Autodesk Fusion 360 part; units mm, degrees
note: some values were not read from the file. Set by a fixed rule: which face or edge a step refers to.
(part 2 of 2)
sketch "Sketch12" plane through (0, 3, 0) normal (0, 1, 0) x (-1, 0, 0) in component "DisplayMount"
  circle A0 centre (-31.9526, 89.8787) radius 5.5
  circle A1 centre (-31.9526, 43.8787) radius 5.5
  circle A2 centre (-230, 35) radius 6.5
  circle A3 centre (-230, 113) radius 6.5
  circle A4 centre (-204.5, 33.25) radius 0.95
  circle A5 centre (-254, 101.75) radius 0.95
  circle A6 centre (-204.5, 101.75) radius 0.95
  circle A7 centre (-254, 33.25) radius 0.95
  line L0 (-205.5, 60.85) -> (-205.5, 66.5)
  line L1 (-205.5, 66.5) -> (-196.5, 66.5)
  line L2 (-196.5, 66.5) -> (-196.5, 60.85)
  line L3 (-196.5, 60.85) -> (-205.5, 60.85)
  line L4 (-205.5, 129.35) -> (-205.5, 135)
  line L5 (-205.5, 135) -> (-196.5, 135)
  line L6 (-196.5, 135) -> (-196.5, 129.35)
  line L7 (-196.5, 129.35) -> (-205.5, 129.35)
  line L8 (-262, 68.5) -> (-262, 74.15)
  line L9 (-262, 74.15) -> (-252.75, 74.15)
  line L10 (-252.75, 74.15) -> (-252.75, 68.5)
  line L11 (-252.75, 68.5) -> (-262, 68.5)
  line L12 (-262, 0) -> (-262, 5.65)
  line L13 (-262, 5.65) -> (-252.75, 5.65)
  line L14 (-252.75, 5.65) -> (-252.75, 0)
  line L15 (-252.75, 0) -> (-262, 0)
  circle A8 centre (-139, 33.25) radius 0.95
  circle A9 centre (-188.5, 101.75) radius 0.95
  circle A10 centre (-139, 101.75) radius 0.95
  line L16 (-140, 60.85) -> (-140, 66.5)
  line L17 (-140, 66.5) -> (-131, 66.5)
  line L18 (-131, 66.5) -> (-131, 60.85)
  line L19 (-131, 60.85) -> (-140, 60.85)
  line L20 (-140, 129.35) -> (-140, 135)
  line L21 (-140, 135) -> (-131, 135)
  line L22 (-131, 135) -> (-131, 129.35)
  line L23 (-131, 129.35) -> (-140, 129.35)
  line L24 (-196.5, 68.5) -> (-196.5, 74.15)
  line L25 (-196.5, 74.15) -> (-187.25, 74.15)
  line L26 (-187.25, 74.15) -> (-187.25, 68.5)
  line L27 (-187.25, 68.5) -> (-196.5, 68.5)
  line L28 (-196.5, 0) -> (-196.5, 5.65)
  line L29 (-196.5, 5.65) -> (-187.25, 5.65)
  line L30 (-187.25, 5.65) -> (-187.25, 0)
  line L31 (-187.25, 0) -> (-196.5, 0)
  circle A11 centre (-73.5, 33.25) radius 0.95
  circle A12 centre (-123, 101.75) radius 0.95
  circle A13 centre (-73.5, 101.75) radius 0.95
  circle A14 centre (-123, 33.25) radius 0.95
  line L32 (-74.5, 60.85) -> (-74.5, 66.5)
  line L33 (-74.5, 66.5) -> (-65.5, 66.5)
  line L34 (-65.5, 66.5) -> (-65.5, 60.85)
  line L35 (-65.5, 60.85) -> (-74.5, 60.85)
  line L36 (-74.5, 129.35) -> (-74.5, 135)
  line L37 (-74.5, 135) -> (-65.5, 135)
  line L38 (-65.5, 135) -> (-65.5, 129.35)
  line L39 (-65.5, 129.35) -> (-74.5, 129.35)
  line L40 (-131, 68.5) -> (-131, 74.15)
  line L41 (-131, 74.15) -> (-121.75, 74.15)
  line L42 (-121.75, 74.15) -> (-121.75, 68.5)
  line L43 (-121.75, 68.5) -> (-131, 68.5)
  line L44 (-131, 0) -> (-131, 5.65)
  line L45 (-131, 5.65) -> (-121.75, 5.65)
  line L46 (-121.75, 5.65) -> (-121.75, 0)
  line L47 (-121.75, 0) -> (-131, 0)
  circle A15 centre (-8, 33.25) radius 0.95
  circle A16 centre (-57.5, 101.75) radius 0.95
  circle A17 centre (-8, 101.75) radius 0.95
  circle A18 centre (-57.5, 33.25) radius 0.95
  line L48 (-9, 60.85) -> (-9, 66.5)
  line L49 (-9, 66.5) -> (0, 66.5)
  line L50 (0, 66.5) -> (0, 60.85)
  line L51 (0, 60.85) -> (-9, 60.85)
  line L52 (-9, 129.35) -> (-9, 135)
  line L53 (-9, 135) -> (0, 135)
  line L54 (0, 135) -> (0, 129.35)
  line L55 (0, 129.35) -> (-9, 129.35)
  line L56 (-65.5, 68.5) -> (-65.5, 74.15)
  line L57 (-65.5, 74.15) -> (-56.25, 74.15)
  line L58 (-56.25, 74.15) -> (-56.25, 68.5)
  line L59 (-56.25, 68.5) -> (-65.5, 68.5)
  line L60 (-65.5, 0) -> (-65.5, 5.65)
  line L61 (-65.5, 5.65) -> (-56.25, 5.65)
  line L62 (-56.25, 5.65) -> (-56.25, 0)
  line L63 (-56.25, 0) -> (-65.5, 0)
  circle A19 centre (-183, 113) radius 6.5
  arc A20 (-188.9673, 32.4229) -> (-189.3593, 33.655) centre (-183, 35) ccw
  arc A21 (-189.3593, 33.655) -> (-188.9673, 32.4229) centre (-188.5, 33.25) ccw
  circle A22 centre (-97.9526, 43.8787) radius 5.5
  circle A23 centre (-97.9526, 89.8787) radius 5.5
  line L64 (1, 89.25) -> (-2, 89.25)
  line L65 (-2, 89.25) -> (-2, 98.75)
  arc A24 (-2, 104.75) -> (-2, 98.75) centre (-2, 101.75) ccw
  line L66 (-2, 104.75) -> (-2, 114.25)
  line L67 (-2, 114.25) -> (1, 114.25)
  line L68 (1, 114.25) -> (1, 136)
  line L69 (1, 136) -> (-22, 136)
  line L70 (-22, 136) -> (-22, 133)
  line L71 (-22, 133) -> (-29, 133)
  arc A25 (-35, 133) -> (-29, 133) centre (-32, 133) ccw
  line L72 (-35, 133) -> (-42, 133)
  line L73 (-42, 133) -> (-42, 136)
  line L74 (-42, 136) -> (-88, 136)
  line L75 (-88, 136) -> (-88, 133)
  line L76 (-88, 133) -> (-95, 133)
  arc A26 (-101, 133) -> (-95, 133) centre (-98, 133) ccw
  line L77 (-101, 133) -> (-108, 133)
  line L78 (-108, 133) -> (-108, 136)
  line L79 (-108, 136) -> (-154, 136)
  line L80 (-154, 136) -> (-154, 133)
  line L81 (-154, 133) -> (-161, 133)
  arc A27 (-167, 133) -> (-161, 133) centre (-164, 133) ccw
  line L82 (-167, 133) -> (-174, 133)
  line L83 (-174, 133) -> (-174, 136)
  line L84 (-174, 136) -> (-220, 136)
  line L85 (-220, 136) -> (-220, 133)
  line L86 (-220, 133) -> (-227, 133)
  arc A28 (-233, 133) -> (-227, 133) centre (-230, 133) ccw
  line L87 (-233, 133) -> (-240, 133)
  line L88 (-240, 133) -> (-240, 136)
  line L89 (-240, 136) -> (-263, 136)
  line L90 (-263, 136) -> (-263, 114.25)
  line L91 (-263, 114.25) -> (-260, 114.25)
  line L92 (-260, 114.25) -> (-260, 104.75)
  arc A29 (-260, 98.75) -> (-260, 104.75) centre (-260, 101.75) ccw
  line L93 (-260, 98.75) -> (-260, 89.25)
  line L94 (-260, 89.25) -> (-263, 89.25)
  line L95 (-263, 89.25) -> (-263, 45.75)
  line L96 (-263, 45.75) -> (-260, 45.75)
  line L97 (-260, 45.75) -> (-260, 36.25)
  arc A30 (-260, 30.25) -> (-260, 36.25) centre (-260, 33.25) ccw
  line L98 (-260, 30.25) -> (-260, 20.75)
  line L99 (-260, 20.75) -> (-263, 20.75)
  line L100 (-263, 20.75) -> (-263, -1)
  line L101 (-263, -1) -> (-240, -1)
  line L102 (-240, -1) -> (-240, 2)
  line L103 (-240, 2) -> (-233, 2)
  arc A31 (-227, 2) -> (-233, 2) centre (-230, 2) ccw
  line L104 (-227, 2) -> (-220, 2)
  line L105 (-220, 2) -> (-220, -1)
  line L106 (-220, -1) -> (-174, -1)
  line L107 (-174, -1) -> (-174, 2)
  line L108 (-174, 2) -> (-167, 2)
  arc A32 (-161, 2) -> (-167, 2) centre (-164, 2) ccw
  line L109 (-161, 2) -> (-154, 2)
  line L110 (-154, 2) -> (-154, -1)
  line L111 (-154, -1) -> (-108, -1)
  line L112 (-108, -1) -> (-108, 2)
  line L113 (-108, 2) -> (-101, 2)
  arc A33 (-95, 2) -> (-101, 2) centre (-98, 2) ccw
  line L114 (-95, 2) -> (-88, 2)
  line L115 (-88, 2) -> (-88, -1)
  line L116 (-88, -1) -> (-42, -1)
  line L117 (-42, -1) -> (-42, 2)
  line L118 (-42, 2) -> (-35, 2)
  arc A34 (-29, 2) -> (-35, 2) centre (-32, 2) ccw
  line L119 (-29, 2) -> (-22, 2)
  line L120 (-22, 2) -> (-22, -1)
  line L121 (-22, -1) -> (1, -1)
  line L122 (1, -1) -> (1, 20.75)
  line L123 (1, 20.75) -> (-2, 20.75)
  line L124 (-2, 20.75) -> (-2, 30.25)
  arc A35 (-2, 36.25) -> (-2, 30.25) centre (-2, 33.25) ccw
  line L125 (-2, 36.25) -> (-2, 45.75)
  line L126 (-2, 45.75) -> (1, 45.75)
  line L127 (1, 45.75) -> (1, 89.25)
  circle A36 centre (-254, 101.75) radius 0.95
  circle A37 centre (-8, 101.75) radius 0.95
  circle A38 centre (-8, 33.25) radius 0.95
  circle A39 centre (-254, 33.25) radius 0.95
extrude "Extrude18" add sketch "Sketch12" against normal blind 0.1 contours A5 A36 | A7 A39 | A15 A38 | A17 A37 bodies 9 in component "DisplayMount"
chamfer "Chamfer1" distance 9.5 angle 45 12 edges at (257, 3, 101.75) (230, 3, 130) (164, 3, 130) (98, 3, 130) (32, 3, 130) (5, 3, 101.75) (5, 3, 33.25) (32, 3, 5) (98, 3, 5) (164, 3, 5) (230, 3, 5) (257, 3, 33.25) on bodies 9 in component "DisplayMount"
sketch "Sketch13" plane through (0, 0, 0) normal (0, -1, 0) x (1, 0, 0) in component "DisplayMount"
  circle A0 centre (204.5, 33.25) radius 0.95
  circle A1 centre (254, 101.75) radius 0.95
  circle A2 centre (204.5, 101.75) radius 0.95
  circle A3 centre (254, 33.25) radius 0.95
  line L0 (205.5, 66.5) -> (205.5, 60.85)
  line L1 (205.5, 60.85) -> (196.5, 60.85)
  line L2 (196.5, 60.85) -> (196.5, 66.5)
  line L3 (196.5, 66.5) -> (205.5, 66.5)
  line L4 (205.5, 135) -> (205.5, 129.35)
  line L5 (205.5, 129.35) -> (196.5, 129.35)
  line L6 (196.5, 129.35) -> (196.5, 135)
  line L7 (196.5, 135) -> (205.5, 135)
  line L8 (262, 74.15) -> (262, 68.5)
  line L9 (262, 68.5) -> (252.75, 68.5)
  line L10 (252.75, 68.5) -> (252.75, 74.15)
  line L11 (252.75, 74.15) -> (262, 74.15)
  line L12 (262, 5.65) -> (262, 0)
  line L13 (262, 0) -> (252.75, 0)
  line L14 (252.75, 0) -> (252.75, 5.65)
  line L15 (252.75, 5.65) -> (262, 5.65)
  circle A4 centre (139, 33.25) radius 0.95
  circle A5 centre (188.5, 101.75) radius 0.95
  circle A6 centre (139, 101.75) radius 0.95
  circle A7 centre (188.5, 33.25) radius 0.95
  line L16 (140, 66.5) -> (140, 60.85)
  line L17 (140, 60.85) -> (131, 60.85)
  line L18 (131, 60.85) -> (131, 66.5)
  line L19 (131, 66.5) -> (140, 66.5)
  line L20 (140, 135) -> (140, 129.35)
  line L21 (140, 129.35) -> (131, 129.35)
  line L22 (131, 129.35) -> (131, 135)
  line L23 (131, 135) -> (140, 135)
  line L24 (196.5, 74.15) -> (196.5, 68.5)
  line L25 (196.5, 68.5) -> (187.25, 68.5)
  line L26 (187.25, 68.5) -> (187.25, 74.15)
  line L27 (187.25, 74.15) -> (196.5, 74.15)
  line L28 (196.5, 5.65) -> (196.5, 0)
  line L29 (196.5, 0) -> (187.25, 0)
  line L30 (187.25, 0) -> (187.25, 5.65)
  line L31 (187.25, 5.65) -> (196.5, 5.65)
  circle A8 centre (73.5, 33.25) radius 0.95
  circle A9 centre (123, 101.75) radius 0.95
  circle A10 centre (73.5, 101.75) radius 0.95
  circle A11 centre (123, 33.25) radius 0.95
  line L32 (74.5, 66.5) -> (74.5, 60.85)
  line L33 (74.5, 60.85) -> (65.5, 60.85)
  line L34 (65.5, 60.85) -> (65.5, 66.5)
  line L35 (65.5, 66.5) -> (74.5, 66.5)
  line L36 (74.5, 135) -> (74.5, 129.35)
  line L37 (74.5, 129.35) -> (65.5, 129.35)
  line L38 (65.5, 129.35) -> (65.5, 135)
  line L39 (65.5, 135) -> (74.5, 135)
  line L40 (131, 74.15) -> (131, 68.5)
  line L41 (131, 68.5) -> (121.75, 68.5)
  line L42 (121.75, 68.5) -> (121.75, 74.15)
  line L43 (121.75, 74.15) -> (131, 74.15)
  line L44 (131, 5.65) -> (131, 0)
  line L45 (131, 0) -> (121.75, 0)
  line L46 (121.75, 0) -> (121.75, 5.65)
  line L47 (121.75, 5.65) -> (131, 5.65)
  circle A12 centre (8, 33.25) radius 0.95
  circle A13 centre (57.5, 101.75) radius 0.95
  circle A14 centre (8, 101.75) radius 0.95
  circle A15 centre (57.5, 33.25) radius 0.95
  line L48 (9, 66.5) -> (9, 60.85)
  line L49 (9, 60.85) -> (0, 60.85)
  line L50 (0, 60.85) -> (0, 66.5)
  line L51 (0, 66.5) -> (9, 66.5)
  line L52 (9, 135) -> (9, 129.35)
  line L53 (9, 129.35) -> (0, 129.35)
  line L54 (0, 129.35) -> (0, 135)
  line L55 (0, 135) -> (9, 135)
  line L56 (65.5, 74.15) -> (65.5, 68.5)
  line L57 (65.5, 68.5) -> (56.25, 68.5)
  line L58 (56.25, 68.5) -> (56.25, 74.15)
  line L59 (56.25, 74.15) -> (65.5, 74.15)
  line L60 (65.5, 5.65) -> (65.5, 0)
  line L61 (65.5, 0) -> (56.25, 0)
  line L62 (56.25, 0) -> (56.25, 5.65)
  line L63 (56.25, 5.65) -> (65.5, 5.65)
  line L64 (263, -1) -> (263, 136)
  line L65 (263, 136) -> (-1, 136)
  line L66 (-1, 136) -> (-1, -1)
  line L67 (-1, -1) -> (263, -1)
  circle A16 centre (8, 101.75) radius 0.95
  circle A17 centre (254, 101.75) radius 0.95
  circle A18 centre (254, 33.25) radius 0.95
  circle A19 centre (8, 33.25) radius 0.95
extrude "Extrude19" cut sketch "Sketch13" against normal blind 5 contours A1 A17 | A3 A18 | A12 A19 | A14 A16 bodies 9 in component "DisplayMount"
move_face "OffsetFaces2" offset -5 64 faces at (9, 2, 131.2333) (3, 1, 129.35) (74.5, 2, 131.2333) (68.5, 1, 129.35) (140, 2, 131.2333) (134, 1, 129.35) (205.5, 2, 131.2333) (199.5, 1, 129.35) (202.5, 2, 135) (196.5, 2, 133.1167) (131, 2, 133.1167) (137, 2, 135) (71.5, 2, 135) (65.5, 2, 133.1167) (0, 2, 133.1167) (6, 2, 135) (252.75, 2, 72.2667) (187.25, 2, 72.2667) (196.5, 2, 64.6167) (121.75, 2, 72.2667) (131, 2, 64.6167) (56.25, 2, 72.2667) (65.5, 2, 64.6167) (196.5, 2, 70.3833) (262, 2, 70.3833) (205.5, 2, 62.7333) (190.3333, 2, 68.5) (199.5, 2, 60.85) (255.8333, 2, 68.5) (134, 2, 60.85) (124.8333, 2, 68.5) (193.4167, 1, 74.15) (202.5, 2, 66.5) (127.9167, 1, 74.15) (137, 2, 66.5) (140, 2, 62.7333) (258.9167, 1, 74.15) (62.4167, 2, 74.15) (71.5, 2, 66.5) (65.5, 2, 70.3833) (59.3333, 2, 68.5) (68.5, 2, 60.85) (74.5, 2, 62.7333) (6, 2, 66.5) (0, 2, 64.6167) (9, 2, 62.7333) (3, 2, 60.85) (65.5, 2, 1.8833) (131, 2, 1.8833) (196.5, 2, 1.8833) (262, 2, 1.8833) (131, 2, 70.3833) (59.3333, 2, 0) (124.8333, 2, 0) (56.25, 2, 3.7667) (62.4167, 2, 5.65) (127.9167, 1, 5.65) (121.75, 2, 3.7667) (193.4167, 1, 5.65) (187.25, 2, 3.7667) (190.3333, 2, 0) (255.8333, 2, 0) (252.75, 2, 3.7667) (258.9167, 1, 5.65) on bodies 9 in component "DisplayMount"
sketch "Sketch10" plane through (0, 3, 0) normal (0, 1, 0) x (-1, 0, 0) in component "DisplayMount"
  line L0 (-112.5, -1) -> (-149.5, -1)
  line L1 (-149.5, -1) -> (-149.5, 136)
  line L2 (-149.5, 136) -> (-112.5, 136)
  line L3 (-112.5, 136) -> (-112.5, -1)
  line L4 (-112.5, -1) -> (-149.5, 136) construction
  line L5 (-149.5, -1) -> (-112.5, 136) construction
  line L6 (-151.8653, 136) -> (-110.1347, 136) construction
  circle A0 centre (-139, 33.25) radius 0.95
  circle A1 centre (-123, 33.25) radius 0.95
  circle A2 centre (-139, 101.75) radius 0.95
  circle A3 centre (-123, 101.75) radius 0.95
  line L7 (-126, 124.35) -> (-145, 124.35)
  line L8 (-145, 124.35) -> (-145, 136)
  line L9 (-126, 136) -> (-126, 124.35)
  circle A4 centre (-139, 101.75) radius 0.95
  circle A5 centre (-123, 101.75) radius 0.95
  line L10 (-136, 71.5) -> (-136, 79.15)
  line L11 (-136, 79.15) -> (-116.75, 79.15)
  line L12 (-116.75, 79.15) -> (-116.75, 63.5)
  line L13 (-116.75, 63.5) -> (-126, 63.5)
  line L14 (-126, 63.5) -> (-126, 55.85)
  line L15 (-126, 55.85) -> (-145, 55.85)
  line L16 (-145, 55.85) -> (-145, 71.5)
  line L17 (-145, 71.5) -> (-136, 71.5)
  circle A6 centre (-139, 33.25) radius 0.95
  circle A7 centre (-123, 33.25) radius 0.95
  line L18 (-136, 10.65) -> (-116.75, 10.65)
  line L19 (-136, -1) -> (-136, 10.65)
  line L20 (-116.75, 10.65) -> (-116.75, -1)
  line L21 (-151.8653, -1) -> (-136, -1)
  point P0 (-131, 67.5)
  point P1 (-151.8653, 136)
  point P2 (-110.1347, 136)
  dimension "d279" = 37
  constraint horizontal L0
  constraint perpendicular L0 L1
  constraint parallel L0 L2
  constraint parallel L1 L3
  constraint coincident L4 P0
  constraint coincident L5 P0
  constraint midpoint L2 L6
  constraint horizontal L6
  constraint coincident P1 L6.start
  constraint coincident P2 L6.end
  constraint collinear L0 L21
  measures "d279" distance of L1.end L2.end
extrude "Extrude14" add sketch "Sketch10" along normal blind 2 separate body contours L0 L1 L2 L3 L7 L8 L9 L18 L19 L20 L21 makes body 11 in component "DisplayMount"
ref_plane "WorkPlane1" through (131, 1.5, 67.5) normal (-1, 0, 0) x (0, 0, 1) in component "DisplayMount"
split "Split1" by plane through (131, 1.5, 67.5) normal (-1, 0, 0) bodies 9 makes body 12 at (19.6406, 0, 14.0761) in component "DisplayMount"
sketch "Sketch1 (2)" plane through (-1, 0, 0) normal (1, 0, 0) x (0, 1, 0) in component "Enclosure"
  line L0 (0, 136) -> (49, 136) construction
  line L1 (49, 136) -> (49, -1) construction
  line L2 (49, -1) -> (0, -1) construction
  line L3 (-3, 140.2) -> (53.2, 140.2)
  line L4 (53.2, 140.2) -> (53.2, -5.2)
  line L5 (53.2, -5.2) -> (-3, -5.2)
  line L6 (-3, 140.2) -> (-3, -5.2) construction
  line L7 (-5.2, 140.2) -> (-5.2, -5.2)
  line L8 (-5.2, 140.2) -> (-3, 140.2)
  line L9 (-3, -5.2) -> (-5.2, -5.2)
  line L10 (3, -1) -> (0, -1)
  line L11 (-3, 74.15) -> (-3, 69.15)
  line L12 (49, 45.75) -> (49, 20.75)
  line L13 (0, 55.85) -> (3, 55.85)
  line L14 (0, -1) -> (0, 55.85)
  line L15 (3, 55.85) -> (3, 45.75)
  line L16 (3, 45.75) -> (49, 45.75)
  line L17 (49, 20.75) -> (3, 20.75)
  line L18 (3, 20.75) -> (3, -1)
  point P0 (49, -1)
  point P1 (0, 136)
  point P2 (49, 136)
  dimension "d184" = 2.2
  constraint coincident P0 L1.end
  constraint perpendicular L5 L6
  constraint perpendicular L6 L8
  constraint equal L6 L7
  constraint horizontal L0
  constraint horizontal L2
  constraint collinear L6 L11
  constraint coincident L0.end L1.start
  constraint coincident P1 L0.start
extrude "Extrude1''" add sketch "Sketch1 (2)" against normal blind 4.2 separate body contours L3 L4 L5 L7 L8 L9 | L10 L12 L13 L14 L15 L16 L17 L18 makes body 13 in component "Enclosure"
sketch "Sketch2 (3)" plane through (-5.2, 0, 0) normal (-1, 0, 0) x (0, -1, 0) in component "Enclosure"
  line L0 (5.2, -5.2) -> (5.2, 140.2)
  line L1 (5.2, 140.2) -> (-53.2, 140.2)
  line L2 (-53.2, 140.2) -> (-53.2, -5.2)
  line L3 (-53.2, -5.2) -> (5.2, -5.2)
  line L4 (-53.2, 140.2) -> (5.2, 140.2)
  line L5 (5.2, 136) -> (-53.2, 136)
  line L6 (-53.2, 136) -> (-53.2, 140.2)
  line L7 (-33.7333, 136) -> (-33.7333, 140.2)
  line L8 (-14.2667, 136) -> (-14.2667, 140.2)
  line L9 (-53.2, 140.2) -> (-49, 140.2)
  line L10 (-49, 140.2) -> (-49, -5.2)
  line L11 (-49, -5.2) -> (-53.2, -5.2)
  line L12 (-53.2, -5.2) -> (-53.2, 140.2)
  line L13 (-53.2, 111.12) -> (-49, 111.12)
  line L14 (-53.2, 82.04) -> (-49, 82.04)
  line L15 (-53.2, 52.96) -> (-49, 52.96)
  line L16 (-53.2, 23.88) -> (-49, 23.88)
  line L17 (-53.2, -5.2) -> (-49, -5.2)
  line L18 (5.2, -5.2) -> (5.2, 140.2) construction
  line L19 (5.2, 67.5) -> (-53.2, 67.5)
  line L20 (5.2, -1) -> (-53.2, -1)
  line L21 (-53.2, -5.2) -> (5.2, -5.2)
  line L22 (-33.7333, -1) -> (-33.7333, -5.2)
  line L23 (-14.2667, -1) -> (-14.2667, -5.2)
  line L24 (5.2, -5.2) -> (5.2, -1)
  line L25 (-53.2, -1) -> (-53.2, -5.2)
  point P0 (-53.2, 140.2)
  dimension "d187" = 4.2
  dimension "d190" = 58.4
  dimension "d191" = 0
  dimension "d192" = 4.2
  dimension "d195" = 0
  dimension "d196" = -145.4
  constraint horizontal L4
  constraint horizontal L5
  constraint vertical L6
  constraint coincident P0 L1.end
  constraint horizontal L9
  constraint vertical L10
  constraint horizontal L11
  constraint vertical L12
  constraint collinear L3 L11
  constraint midpoint L18 L19.start
  constraint midpoint L12 L19.end
  constraint symmetric P0 L19 L2.end
  constraint symmetric L5.start L19 L20.start
  constraint symmetric L5.end L19 L20.end
  constraint symmetric L7.start L19 L22.start
  constraint symmetric L7.end L19 L22.end
  constraint symmetric L8.start L19 L23.start
  constraint symmetric L8.end L19 L23.end
  constraint coincident L0.end L1.start
  constraint coincident L5.start L18
  constraint coincident L0.start L3.end
  measures "d187" distance of P0 L5.end
  measures "d192" distance of P0 L9.end
extrude "Extrude2'" cut sketch "Sketch2 (3)" against normal up to surface (4.2 mm away) contours L3 L20 L21 L22 L23 | L1 L4 L5 L7 L8 | L2 L10 L12 L13 L14 | L2 L10 L12 L15 L16 bodies 13 in component "Enclosure"
ref_plane "WorkPlane1" through (131, 24.5, 97.925) normal (-1, 0, 0) x (0, 0, 1) in component "Enclosure"
ref_plane "WorkPlane2" through (102.75, 24.5, 67.5) normal (0, 0, 1) x (1, 0, 0) in component "Enclosure"
mirror "Mirror1" about plane through (131, 24.5, 97.925) normal (-1, 0, 0) of bodies 13 makes body 14 in component "Enclosure"
sketch "Sketch3 (2)" plane through (0, 0, 140.2) normal (0, 0, 1) x (-1, 0, 0) in component "Enclosure"
  line L0 (-267.2, -14.2667) -> (-263, -14.2667)
  line L1 (-263, -14.2667) -> (-263, 5.2)
  line L2 (-263, 5.2) -> (-267.2, 5.2)
  line L3 (-267.2, 5.2) -> (-267.2, -14.2667)
  line L4 (-267.2, 5.2) -> (5.2, 5.2)
  line L5 (5.2, 5.2) -> (5.2, -53.2)
  line L6 (5.2, -53.2) -> (-267.2, -53.2)
  line L7 (-267.2, -53.2) -> (-267.2, 5.2)
  point P0 (-267.2, 5.2)
  point P1 (5.2, -53.2)
  constraint horizontal L4
  constraint vertical L5
  constraint horizontal L6
  constraint vertical L7
  constraint coincident P1 L5.end
  constraint coincident P0 L2.end
extrude "Extrude3''" add sketch "Sketch3 (2)" against normal blind 4.2 separate body contours L0 L1 L4 L5 L6 L7 makes body 15 in component "Enclosure"
combine "Combine1" operation cut target body 15 tool bodies 14 13 keep tools in component "Enclosure"
sketch "Sketch4 (2)" plane through (0, 0, 140.2) normal (0, 0, 1) x (-1, 0, 0) in component "Enclosure"
  line L0 (-263, -33.7333) -> (-263, -53.2)
  line L1 (-263, -53.2) -> (1, -53.2)
  line L2 (5.2, -33.7333) -> (5.2, -14.2667)
  line L3 (1, 5.2) -> (-263, 5.2)
  line L4 (-263, 5.2) -> (-263, -14.2667)
  line L5 (-263, -14.2667) -> (-267.2, -14.2667)
  line L6 (-267.2, -14.2667) -> (-267.2, -33.7333)
  line L7 (-267.2, -33.7333) -> (-263, -33.7333)
  line L8 (-263, -53.2) -> (1, -53.2)
  line L9 (1, -53.2) -> (1, -49)
  line L10 (1, -49) -> (-263, -49)
  line L11 (-263, -49) -> (-263, -53.2)
  line L12 (-225.2857, -49) -> (-225.2857, -53.2)
  line L13 (-187.5714, -49) -> (-187.5714, -53.2)
  line L14 (-149.8571, -49) -> (-149.8571, -53.2)
  line L15 (-112.1429, -49) -> (-112.1429, -53.2)
  line L16 (-74.4286, -49) -> (-74.4286, -53.2)
  line L17 (-36.7143, -49) -> (-36.7143, -53.2)
  line L18 (1, -49) -> (1, -53.2)
  line L19 (1, -14.2667) -> (1, 5.2)
  line L20 (1, -53.2) -> (1, -33.7333)
  line L21 (1, -33.7333) -> (5.2, -33.7333)
  line L22 (5.2, -14.2667) -> (1, -14.2667)
  point P0 (-263, -53.2)
  dimension "d205" = 4.2
  dimension "d208" = 264
  dimension "d209" = 0
  constraint horizontal L8
  constraint vertical L9
  constraint horizontal L10
  constraint vertical L11
  constraint coincident P0 L0.end
  constraint collinear L9 L20
  measures "d205" distance of P0 L10.end
extrude "Extrude4'" cut sketch "Sketch4 (2)" against normal up to surface (4.2 mm away) contours L1 L8 L10 L12 L13 | L1 L8 L10 L14 L15 | L1 L8 L10 L16 L17 bodies 15 in component "Enclosure"
mirror "Mirror2" about plane through (102.75, 24.5, 67.5) normal (0, 0, 1) of bodies 15 makes body 16 in component "Enclosure"
sketch "Sketch3 (3)" plane through (0, 53.2, 0) normal (0, 1, 0) x (-1, 0, 0) in component "Enclosure"
  line L0 (-267.2, 111.12) -> (-263, 111.12)
  line L1 (-263, 111.12) -> (-263, 140.2)
  line L2 (-263, 140.2) -> (-267.2, 140.2)
  line L3 (-267.2, 140.2) -> (-267.2, 111.12)
  line L4 (-267.2, 140.2) -> (5.2, 140.2)
  line L5 (5.2, 140.2) -> (5.2, -5.2)
  line L6 (5.2, -5.2) -> (-267.2, -5.2)
  line L7 (-267.2, -5.2) -> (-267.2, 140.2)
  point P0 (-267.2, 140.2)
  point P1 (5.2, -5.2)
  constraint horizontal L4
  constraint vertical L5
  constraint horizontal L6
  constraint vertical L7
  constraint coincident P1 L5.end
  constraint coincident P0 L2.end
extrude "Extrude5" add sketch "Sketch3 (3)" against normal blind 4.2 separate body contours L0 L1 L4 L5 L6 L7 makes body 17 in component "Enclosure"
combine "Combine2" operation cut target body 17 tool bodies 15 14 13 16 keep tools in component "Enclosure"
sketch "Sketch5" plane through (0, 53.2, 0) normal (0, 1, 0) x (-1, 0, 0) in component "Enclosure"
  line L0 (-263, -1) -> (-225.2857, -1)
  line L1 (-225.2857, -1) -> (-225.2857, -5.2)
  line L2 (-225.2857, -5.2) -> (-187.5714, -5.2)
  line L3 (-187.5714, -5.2) -> (-187.5714, -1)
  line L4 (-187.5714, -1) -> (-149.8571, -1)
  line L5 (-149.8571, -1) -> (-149.8571, -5.2)
  line L6 (-112.1429, -5.2) -> (-112.1429, -1)
  line L7 (-112.1429, -1) -> (-74.4286, -1)
  line L8 (-74.4286, -1) -> (-74.4286, -5.2)
  line L9 (-36.7143, -5.2) -> (-36.7143, -1)
  line L10 (-36.7143, -1) -> (1, -1)
  line L11 (1, 23.88) -> (5.2, 23.88)
  line L12 (5.2, 23.88) -> (5.2, 52.96)
  line L13 (5.2, 52.96) -> (1, 52.96)
  line L14 (1, 82.04) -> (5.2, 82.04)
  line L15 (5.2, 82.04) -> (5.2, 111.12)
  line L16 (5.2, 111.12) -> (1, 111.12)
  line L17 (1, 136) -> (-36.7143, 136)
  line L18 (-36.7143, 136) -> (-36.7143, 140.2)
  line L19 (-36.7143, 140.2) -> (-74.4286, 140.2)
  line L20 (-74.4286, 140.2) -> (-74.4286, 136)
  line L21 (-74.4286, 136) -> (-112.1429, 136)
  line L22 (-112.1429, 136) -> (-112.1429, 140.2)
  line L23 (-112.1429, 140.2) -> (-149.8571, 140.2)
  line L24 (-149.8571, 140.2) -> (-149.8571, 136)
  line L25 (-149.8571, 136) -> (-187.5714, 136)
  line L26 (-187.5714, 136) -> (-187.5714, 140.2)
  line L27 (-187.5714, 140.2) -> (-225.2857, 140.2)
  line L28 (-225.2857, 140.2) -> (-225.2857, 136)
  line L29 (-225.2857, 136) -> (-263, 136)
  line L30 (-263, 111.12) -> (-267.2, 111.12)
  line L31 (-267.2, 111.12) -> (-267.2, 82.04)
  line L32 (-267.2, 82.04) -> (-263, 82.04)
  line L33 (-263, 52.96) -> (-267.2, 52.96)
  line L34 (-267.2, 52.96) -> (-267.2, 23.88)
  line L35 (-267.2, 23.88) -> (-263, 23.88)
  line L36 (-194.5, 2) -> (-219.5, 2)
  line L37 (-219.5, 2) -> (-219.5, 13.9)
  line L38 (-219.5, 13.9) -> (-194.5, 13.9)
  line L39 (-194.5, 13.9) -> (-194.5, 2)
  line L40 (-194.5, 2) -> (-219.5, 13.9) construction
  line L41 (-219.5, 2) -> (-194.5, 13.9) construction
  line L42 (-236, 116) -> (-236, 31) construction
  line L43 (-178, 31) -> (-178, 116) construction
  line L44 (-236, 116) -> (-178, 116)
  line L45 (-178, 116) -> (-178, 114.6)
  line L46 (-178, 114.6) -> (-236, 114.6)
  line L47 (-236, 114.6) -> (-236, 116)
  line L48 (-236, 108.9167) -> (-178, 108.9167)
  line L49 (-178, 107.5167) -> (-236, 107.5167)
  line L50 (-236, 107.5167) -> (-236, 108.9167)
  line L51 (-178, 108.9167) -> (-178, 107.5167)
  line L52 (-236, 101.8333) -> (-178, 101.8333)
  line L53 (-178, 100.4333) -> (-236, 100.4333)
  line L54 (-236, 100.4333) -> (-236, 101.8333)
  line L55 (-178, 101.8333) -> (-178, 100.4333)
  line L56 (-236, 94.75) -> (-178, 94.75)
  line L57 (-178, 93.35) -> (-236, 93.35)
  line L58 (-236, 93.35) -> (-236, 94.75)
  line L59 (-178, 94.75) -> (-178, 93.35)
  line L60 (-236, 87.6667) -> (-178, 87.6667)
  line L61 (-178, 86.2667) -> (-236, 86.2667)
  line L62 (-236, 86.2667) -> (-236, 87.6667)
  line L63 (-178, 87.6667) -> (-178, 86.2667)
  line L64 (-236, 80.5833) -> (-178, 80.5833)
  line L65 (-178, 79.1833) -> (-236, 79.1833)
  line L66 (-236, 79.1833) -> (-236, 80.5833)
  line L67 (-178, 80.5833) -> (-178, 79.1833)
  line L68 (-236, 73.5) -> (-178, 73.5)
  line L69 (-178, 72.1) -> (-236, 72.1)
  line L70 (-236, 72.1) -> (-236, 73.5)
  line L71 (-178, 73.5) -> (-178, 72.1)
  line L72 (-236, 66.4167) -> (-178, 66.4167)
  line L73 (-178, 65.0167) -> (-236, 65.0167)
  line L74 (-236, 65.0167) -> (-236, 66.4167)
  line L75 (-178, 66.4167) -> (-178, 65.0167)
  line L76 (-236, 59.3333) -> (-178, 59.3333)
  line L77 (-178, 57.9333) -> (-236, 57.9333)
  line L78 (-236, 57.9333) -> (-236, 59.3333)
  line L79 (-178, 59.3333) -> (-178, 57.9333)
  line L80 (-236, 52.25) -> (-178, 52.25)
  line L81 (-178, 50.85) -> (-236, 50.85)
  line L82 (-236, 50.85) -> (-236, 52.25)
  line L83 (-178, 52.25) -> (-178, 50.85)
  line L84 (-236, 45.1667) -> (-178, 45.1667)
  line L85 (-178, 43.7667) -> (-236, 43.7667)
  line L86 (-236, 43.7667) -> (-236, 45.1667)
  line L87 (-178, 45.1667) -> (-178, 43.7667)
  line L88 (-236, 38.0833) -> (-178, 38.0833)
  line L89 (-178, 36.6833) -> (-236, 36.6833)
  line L90 (-236, 36.6833) -> (-236, 38.0833)
  line L91 (-178, 38.0833) -> (-178, 36.6833)
  line L92 (-236, 31) -> (-178, 31)
  line L93 (-178, 29.6) -> (-236, 29.6)
  line L94 (-236, 29.6) -> (-236, 31)
  line L95 (-178, 31) -> (-178, 29.6)
  circle A0 centre (-230, 133) radius 1.6 construction
  circle A1 centre (-164, 133) radius 1.6 construction
  circle A2 centre (-98, 133) radius 1.6 construction
  circle A3 centre (-32, 133) radius 1.6 construction
  circle A4 centre (-32, 2) radius 1.6 construction
  circle A5 centre (-98, 2) radius 1.6 construction
  circle A6 centre (-164, 2) radius 1.6 construction
  circle A7 centre (-230, 2) radius 1.6 construction
  circle A8 centre (-230, 133) radius 1.1
  circle A9 centre (-164, 133) radius 1.1
  circle A10 centre (-98, 133) radius 1.1
  circle A11 centre (-32, 133) radius 1.1
  circle A12 centre (-2, 101.75) radius 1.1
  circle A13 centre (-32, 2) radius 1.1
  circle A14 centre (-98, 2) radius 1.1
  circle A15 centre (-164, 2) radius 1.1
  circle A16 centre (-230, 2) radius 1.1
  circle A17 centre (-260, 33.25) radius 1.1
  line L96 (1, 52.96) -> (1, 82.04)
  line L97 (1, 111.12) -> (1, 136)
  line L98 (-263, 82.04) -> (-263, 52.96)
  line L99 (-263, 23.88) -> (-263, -1)
  line L100 (1, -1) -> (1, 23.88)
  line L101 (-263, 136) -> (-263, 111.12)
  line L102 (-149.8571, -5.2) -> (-112.1429, -5.2)
  line L103 (-74.4286, -5.2) -> (-36.7143, -5.2)
  circle A18 centre (-260, 101.75) radius 1.6 construction
  circle A19 centre (-260, 101.75) radius 1
  circle A20 centre (-2, 33.25) radius 1.1
  line L104 (-230, 2) -> (-164, 2) construction
  line L105 (-207, 29.6) -> (-207, 2) construction
  circle A21 centre (-2, 101.75) radius 1.6
  circle A22 centre (-260, 33.25) radius 1.6
  circle A23 centre (-2, 33.25) radius 1.6
  point P0 (-207, 7.95)
  dimension "d223" = 11.9
  dimension "d225" = 1.4
  dimension "d228" = 0
  dimension "d229" = -85
  dimension "d230" = 2.2
  dimension "d231" = 2.2
  dimension "d232" = 2.2
  dimension "d233" = 2.2
  dimension "d234" = 2.2
  dimension "d235" = 2.2
  dimension "d236" = 2.2
  dimension "d237" = 2.2
  dimension "d238" = 2.2
  dimension "d239" = 2.2
  dimension "d274" = 2
  dimension "d275" = 2.2
  dimension "d280" = 25
  constraint horizontal L36
  constraint perpendicular L36 L37
  constraint parallel L36 L38
  constraint parallel L37 L39
  constraint coincident L40 P0
  constraint coincident L41 P0
  constraint horizontal L44
  constraint vertical L45
  constraint horizontal L46
  constraint vertical L47
  constraint coincident L43 L45.end
  constraint coincident L42.start L44.start
  constraint concentric A0 A8
  constraint concentric A1 A9
  constraint concentric A2 A10
  constraint concentric A3 A11
  constraint concentric A12 A21
  constraint concentric A4 A13
  constraint concentric A5 A14
  constraint concentric A6 A15
  constraint concentric A7 A16
  constraint concentric A17 A22
  constraint concentric A18 A19
  constraint concentric A20 A23
  constraint coincident A7.centre A16.centre
  constraint coincident A6.centre A15.centre
  constraint midpoint L93 L105.start
  constraint coincident L104 L105.end
  constraint perpendicular L104 L105
  constraint collinear L36 L104
  constraint coincident P0 L105
  measures "d223" distance of L36.end L37.end
  measures "d225" distance of L42.start L46.end
  measures "d230" diameter of A8
  measures "d231" diameter of A9
  measures "d232" diameter of A10
  measures "d233" diameter of A11
  measures "d234" diameter of A12
  measures "d235" diameter of A13
  measures "d236" diameter of A14
  measures "d237" diameter of A15
  measures "d238" diameter of A16
  measures "d239" diameter of A17
  measures "d274" diameter of A19
  measures "d275" diameter of A20
  measures "d280" distance of L37 L39
extrude "PowerConnectorBack" cut sketch "Sketch5" against normal up to surface (4.2 mm away) contours L36 L37 L38 L39 | L52 L53 L54 L55 | L56 L57 L58 L59 | L60 L61 L62 L63 | L64 L65 L66 L67 | L68 L69 L70 L71 | L72 L73 L74 L75 | L76 L77 L78 L79 | L80 L81 L82 L83 | L84 L85 L86 L87 | A8 | A9 | A10 | A11 | A12 | A13 | A14 | A15 | A16 | A17 | A19 | A20 bodies 17 in component "Enclosure"
sketch "Sketch6" plane through (0, 53.2, 0) normal (0, 1, 0) x (-1, 0, 0) in component "Enclosure"
  line L0 (-178, 45.1667) -> (-178, 43.7667)
  line L1 (-178, 43.7667) -> (-236, 43.7667)
  line L2 (-236, 43.7667) -> (-236, 45.1667)
  line L3 (-236, 45.1667) -> (-178, 45.1667)
  line L4 (-178, 73.5) -> (-178, 72.1)
  line L5 (-178, 72.1) -> (-236, 72.1)
  line L6 (-236, 72.1) -> (-236, 73.5)
  line L7 (-236, 73.5) -> (-178, 73.5)
  line L8 (-178, 101.8333) -> (-178, 100.4333)
  line L9 (-178, 100.4333) -> (-236, 100.4333)
  line L10 (-236, 100.4333) -> (-236, 101.8333)
  line L11 (-236, 101.8333) -> (-178, 101.8333)
  line L12 (-178, 94.75) -> (-178, 93.35)
  line L13 (-178, 93.35) -> (-236, 93.35)
  line L14 (-236, 93.35) -> (-236, 94.75)
  line L15 (-236, 94.75) -> (-178, 94.75)
  line L16 (-178, 66.4167) -> (-178, 65.0167)
  line L17 (-178, 65.0167) -> (-236, 65.0167)
  line L18 (-236, 65.0167) -> (-236, 66.4167)
  line L19 (-236, 66.4167) -> (-178, 66.4167)
  circle A0 centre (-2, 101.75) radius 1.1
  line L20 (-178, 52.25) -> (-178, 50.85)
  line L21 (-178, 50.85) -> (-236, 50.85)
  line L22 (-236, 50.85) -> (-236, 52.25)
  line L23 (-236, 52.25) -> (-178, 52.25)
  line L24 (-178, 80.5833) -> (-178, 79.1833)
  line L25 (-178, 79.1833) -> (-236, 79.1833)
  line L26 (-236, 79.1833) -> (-236, 80.5833)
  line L27 (-236, 80.5833) -> (-178, 80.5833)
  line L28 (-194.5, 13.9) -> (-194.5, 2)
  line L29 (-194.5, 2) -> (-219.5, 2)
  line L30 (-219.5, 2) -> (-219.5, 13.9)
  line L31 (-219.5, 13.9) -> (-194.5, 13.9)
  line L32 (-178, 87.6667) -> (-178, 86.2667)
  line L33 (-178, 86.2667) -> (-236, 86.2667)
  line L34 (-236, 86.2667) -> (-236, 87.6667)
  line L35 (-236, 87.6667) -> (-178, 87.6667)
  line L36 (-178, 59.3333) -> (-178, 57.9333)
  line L37 (-178, 57.9333) -> (-236, 57.9333)
  line L38 (-236, 57.9333) -> (-236, 59.3333)
  line L39 (-236, 59.3333) -> (-178, 59.3333)
  circle A1 centre (-260, 33.25) radius 1.1
  line L40 (-263, -1) -> (-225.2857, -1)
  line L41 (-225.2857, -1) -> (-225.2857, -5.2)
  line L42 (-225.2857, -5.2) -> (-187.5714, -5.2)
  line L43 (-187.5714, -5.2) -> (-187.5714, -1)
  line L44 (-187.5714, -1) -> (-149.8571, -1)
  line L45 (-149.8571, -1) -> (-149.8571, -5.2)
  line L46 (-112.1429, -5.2) -> (-112.1429, -1)
  line L47 (-112.1429, -1) -> (-74.4286, -1)
  line L48 (-74.4286, -1) -> (-74.4286, -5.2)
  line L49 (-36.7143, -5.2) -> (-36.7143, -1)
  line L50 (-36.7143, -1) -> (1, -1)
  line L51 (1, -1) -> (1, 23.88)
  line L52 (1, 23.88) -> (5.2, 23.88)
  line L53 (5.2, 23.88) -> (5.2, 52.96)
  line L54 (5.2, 52.96) -> (1, 52.96)
  line L55 (1, 52.96) -> (1, 82.04)
  line L56 (1, 82.04) -> (5.2, 82.04)
  line L57 (5.2, 82.04) -> (5.2, 111.12)
  line L58 (5.2, 111.12) -> (1, 111.12)
  line L59 (1, 111.12) -> (1, 136)
  line L60 (1, 136) -> (-36.7143, 136)
  line L61 (-36.7143, 136) -> (-36.7143, 140.2)
  line L62 (-36.7143, 140.2) -> (-74.4286, 140.2)
  line L63 (-74.4286, 140.2) -> (-74.4286, 136)
  line L64 (-74.4286, 136) -> (-112.1429, 136)
  line L65 (-112.1429, 136) -> (-112.1429, 140.2)
  line L66 (-112.1429, 140.2) -> (-149.8571, 140.2)
  line L67 (-149.8571, 140.2) -> (-149.8571, 136)
  line L68 (-149.8571, 136) -> (-187.5714, 136)
  line L69 (-187.5714, 136) -> (-187.5714, 140.2)
  line L70 (-187.5714, 140.2) -> (-225.2857, 140.2)
  line L71 (-225.2857, 140.2) -> (-225.2857, 136)
  line L72 (-225.2857, 136) -> (-263, 136)
  line L73 (-263, 136) -> (-263, 111.12)
  line L74 (-263, 111.12) -> (-267.2, 111.12)
  line L75 (-267.2, 111.12) -> (-267.2, 82.04)
  line L76 (-267.2, 82.04) -> (-263, 82.04)
  line L77 (-263, 82.04) -> (-263, 52.96)
  line L78 (-263, 52.96) -> (-267.2, 52.96)
  line L79 (-267.2, 52.96) -> (-267.2, 23.88)
  line L80 (-267.2, 23.88) -> (-263, 23.88)
  line L81 (-263, 23.88) -> (-263, -1)
  line L82 (-131, 140.2) -> (-131, 130.2) construction
  circle A2 centre (-131, 130.2) radius 2.6
  line L83 (-128.4, 132.4) -> (-133.6, 132.4)
  line L84 (-133.6, 132.4) -> (-133.6, 128)
  line L85 (-133.6, 128) -> (-128.4, 128)
  line L86 (-128.4, 128) -> (-128.4, 132.4)
  line L87 (-128.4, 132.4) -> (-133.6, 128) construction
  line L88 (-133.6, 132.4) -> (-128.4, 128) construction
  circle A3 centre (-32, 2) radius 1.1
  circle A4 centre (-164, 133) radius 1.1
  circle A5 centre (-98, 133) radius 1.1
  circle A6 centre (-98, 2) radius 1.1
  circle A7 centre (-260, 101.75) radius 1
  circle A8 centre (-230, 2) radius 1.1
  circle A9 centre (-230, 133) radius 1.1
  circle A10 centre (-32, 133) radius 1.1
  circle A11 centre (-164, 2) radius 1.1
  circle A12 centre (-2, 33.25) radius 1.1
  line L89 (-149.8571, -5.2) -> (-112.1429, -5.2)
  line L90 (-74.4286, -5.2) -> (-36.7143, -5.2)
  point P0 (-131, 130.2)
  dimension "d247" = 10
  dimension "d248" = 5.2
  dimension "d249" = 4.4
  constraint vertical L82
  constraint midpoint L66 L82.start
  constraint coincident P0 L82.end
  constraint horizontal L83
  constraint perpendicular L83 L84
  constraint parallel L83 L85
  constraint parallel L84 L86
  constraint coincident L87 P0
  constraint coincident L88 P0
  constraint tangent A2 L84
  measures "d247" distance of L82.start P0
  measures "d248" diameter of A2
  measures "d249" distance of L83.end L84.end
extrude "Extrude7" cut sketch "Sketch6" against normal blind 2.1 contours A2 L83 L85 bodies 17 in component "Enclosure"
sketch "Sketch7" plane through (0, 51.1, 0) normal (0, 1, 0) x (-1, 0, 0) in component "Enclosure"
  arc A0 (-132.3856, 132.4) -> (-132.3856, 128) centre (-131, 130.2) ccw
  line L0 (-132.3856, 128) -> (-129.6144, 128)
  arc A1 (-129.6144, 128) -> (-129.6144, 132.4) centre (-131, 130.2) ccw
  line L1 (-129.6144, 132.4) -> (-132.3856, 132.4)
  line L2 (-131, 132.4) -> (-131, 128) construction
  line L3 (-128.4702, 130.8) -> (-133.5298, 130.8)
  line L4 (-133.5298, 130.8) -> (-133.5298, 129.6)
  line L5 (-133.5298, 129.6) -> (-128.4702, 129.6)
  line L6 (-128.4702, 129.6) -> (-128.4702, 130.8)
  line L7 (-128.4702, 130.8) -> (-133.5298, 129.6) construction
  line L8 (-133.5298, 130.8) -> (-128.4702, 129.6) construction
  point P0 (-131, 130.2)
  dimension "d253" = 1.2
  constraint midpoint L1 L2.start
  constraint midpoint L0 L2.end
  constraint horizontal L3
  constraint perpendicular L3 L4
  constraint parallel L3 L5
  constraint parallel L4 L6
  constraint coincident L7 P0
  constraint coincident L8 P0
  constraint coincident P0 A0.centre
  constraint coincident A0 L3.end
  measures "d253" distance of L3.end L4.end
extrude "Extrude8" cut sketch "Sketch7" against normal up to surface (2.1 mm away) contours L3 L4 L5 L6 bodies 17 in component "Enclosure"
move_face "OffsetFaces1" offset -0.1 20 faces at (225.2857, 50.4, 137.4) (149.8571, 50.4, 137.4) (74.4286, 50.4, 137.4) (265.8, 50.4, 111.12) (187.5714, 50.4, 137.4) (112.1429, 50.4, 137.4) (36.7143, 50.4, 137.4) (-3.8, 51.8, 111.12) (-3.8, 51.8, 52.96) (-3.8, 51.8, 82.04) (-3.8, 51.8, 23.88) (36.7143, 50.4, -2.4) (74.4286, 50.4, -2.4) (149.8571, 50.4, -2.4) (225.2857, 50.4, -2.4) (265.8, 51.8, 23.88) (112.1429, 50.4, -2.4) (187.5714, 50.4, -2.4) (265.8, 51.8, 82.04) (265.8, 51.8, 52.96) on bodies 17 in component "Enclosure"
sketch "Sketch1 (3)" plane through (0, -5.2, 0) normal (0, -1, 0) x (1, 0, 0) in component "FrontGlass"
  line L0 (-1, -5.2) -> (-1, 140.2)
  line L1 (-1, 140.2) -> (-5.2, 140.2)
  line L2 (-5.2, 140.2) -> (-5.2, -5.2)
  line L3 (-5.2, -5.2) -> (-1, -5.2)
  line L4 (-1, 140.2) -> (-1, -5.2) construction
  line L5 (263, 136) -> (-1, 136) construction
  line L6 (263, 140.2) -> (263, -5.2) construction
  line L7 (263, -1) -> (-1, -1) construction
  line L8 (-1, 136) -> (263, 136)
  line L9 (263, 136) -> (263, -1)
  line L10 (263, -1) -> (-1, -1)
  line L11 (-1, -1) -> (-1, 136)
  point P0 (-1, 136)
  constraint horizontal L8
  constraint vertical L9
  constraint horizontal L10
  constraint vertical L11
  constraint coincident L7.start L9.end
  constraint coincident P0 L5.end
extrude "Extrude1'''" add sketch "Sketch1 (3)" against normal up to surface (2.2 mm away) separate body contours L0 L8 L9 L10 L11 makes body 18 in component "FrontGlass"
fillet "Fillet1" radius 2.2 4 edges at (-1, -4.1, 136) (263, -4.1, 136) (263, -4.1, -1) (-1, -4.1, -1) on bodies 18 in component "FrontGlass"
move_face "OffsetFaces2'" offset -0.1 4 faces at (265.8, 33.7333, 137.4) (265.8, 14.2667, 138.8) (-3.8, 33.7333, 137.4) (-3.8, 14.2667, 137.4) on bodies 15 in component "Enclosure"
move_face "OffsetFaces3" offset -0.1 4 faces at (265.8, 33.7333, -2.4) (265.8, 14.2667, -2.4) (-3.8, 33.7333, -2.4) (-3.8, 14.2667, -2.4) on bodies 16 in component "Enclosure"
component "Display" placed x (1, 0, 0) y (0, 1, 0) z (0, 0, 1) at (0, 0, 0)
component "DisplayMount" placed x (1, 0, 0) y (0, 1, 0) z (0, 0, 1) at (0, 0, 0)
component "PowerSupply" placed x (1, 0, 0) y (0, 1, 0) z (0, 0, 1) at (0, 0, 0)
component "Enclosure" placed x (1, 0, 0) y (0, 1, 0) z (0, 0, 1) at (0, 0, 0)
component "FrontGlass" placed x (1, 0, 0) y (0, 1, 0) z (0, 0, 1) at (0, 0, 0)
equation "DisplayModuleWidth = 65.5 mm"
equation "DisplayModuleHeight = 66.5 mm"
equation "d3 = DisplayModuleWidth"
equation "d4 = DisplayModuleHeight"
equation "d11 = 5 mm + 3.2 mm"
equation "d12 = 5 mm + 3.6 mm"
equation "d27 = DisplayModuleWidth"
equation "d28 = DisplayModuleHeight + 2 mm"
equation "d66 = -DisplayModuleWidth"
equation "DisplayMaskThickness = 0.6 mm"
equation "PlywoodThickness = 4.2 mm"
equation "FrontGlassThickness = 2.2 mm"
equation "d184 = FrontGlassThickness"
equation "d185 = -PlywoodThickness"
equation "d187 = PlywoodThickness"
equation "d192 = PlywoodThickness"
equation "d201 = -PlywoodThickness"
equation "d205 = PlywoodThickness"
equation "d212 = -PlywoodThickness"
equation "d225 = PlywoodThickness / 3"
equation "d250 = -PlywoodThickness / 2"
equation "d282 = FrontGlassThickness"
equation "plywoodTolerance = 0.1 mm"
equation "d284 = -plywoodTolerance"
equation "d285 = -plywoodTolerance"
equation "d286 = -plywoodTolerance"
named bodies: "Body1", "Body1 (1)", "Body1 (2)", "Body1 (3)", "Body1 (4)", "Body1 (5)", "Body1 (6)", "Body1 (7)", "DisplayMountRight", "DisplayMountLeft", "EnclosureLeft", "EnclosurRight", "EnclosureTop", "EnclosureBottom", "EnclosureBack"
